Autodesk Fusion 360 part; units mm, degrees
note: some values were not read from the file. Set by a fixed rule: which sketch regions a step uses.
(part 46 of 59)
  spline S74 degree 5 poles (30.2174, 19.4214) (30.2148, 19.4218) (30.2094, 19.4225) (30.2014, 19.4236) (30.1907, 19.425) (30.1773, 19.4267) (30.164, 19.4284) (30.1507, 19.4301) (30.1375, 19.4317) (30.1242, 19.4334) (30.111, 19.435) (30.0979, 19.4366) (30.0847, 19.4382) (30.0716, 19.4398) (30.0585, 19.4413) (30.0455, 19.4428) (30.0324, 19.4443) (30.0194, 19.4458) (30.0065, 19.4473) (29.9935, 19.4487) (29.9806, 19.4501) (29.9678, 19.4516) (29.9549, 19.4529) (29.9421, 19.4543) (29.9293, 19.4556) (29.9166, 19.457) (29.9039, 19.4583) (29.8912, 19.4596) (29.8785, 19.4608) (29.8659, 19.4621) (29.8533, 19.4633) (29.8407, 19.4645) (29.8282, 19.4657) (29.8157, 19.4669) (29.8032, 19.468) (29.7908, 19.4691) (29.7784, 19.4702) (29.766, 19.4713) (29.7537, 19.4724) (29.7414, 19.4735) (29.7291, 19.4745) (29.7169, 19.4755) (29.7047, 19.4765) (29.6925, 19.4775) (29.6803, 19.4784) (29.6682, 19.4794) (29.6562, 19.4803) (29.6441, 19.4812) (29.6321, 19.4821) (29.6201, 19.483) (29.6082, 19.4838) (29.5963, 19.4846) (29.5844, 19.4855) (29.5726, 19.4863) (29.5608, 19.487) (29.549, 19.4878) (29.5373, 19.4885) (29.5256, 19.4892) (29.514, 19.49) (29.5023, 19.4906) (29.4907, 19.4913) (29.4792, 19.492) (29.4677, 19.4926) (29.4562, 19.4932) (29.4447, 19.4938) (29.4333, 19.4944) (29.422, 19.495) (29.4106, 19.4955) (29.3993, 19.496) (29.3881, 19.4965) (29.3768, 19.497) (29.3657, 19.4975) (29.3545, 19.498) (29.3434, 19.4984) (29.3323, 19.4989) (29.3213, 19.4993) (29.3103, 19.4997) (29.2993, 19.5001) (29.2884, 19.5004) (29.2775, 19.5008) (29.2667, 19.5011) (29.2559, 19.5014) (29.2451, 19.5017) (29.2344, 19.502) (29.2237, 19.5023) (29.213, 19.5025) (29.2024, 19.5028) (29.1919, 19.503) (29.1813, 19.5032) (29.1708, 19.5034) (29.1604, 19.5035) (29.15, 19.5037) (29.1396, 19.5038) (29.1293, 19.504) (29.119, 19.5041) (29.1088, 19.5042) (29.0986, 19.5043) (29.0884, 19.5043) (29.0783, 19.5044) (29.0682, 19.5044) (29.0582, 19.5045) (29.0482, 19.5045) (29.0383, 19.5045) (29.0284, 19.5045) (29.0185, 19.5044) (29.0087, 19.5044) (28.9989, 19.5043) (28.9892, 19.5043) (28.9795, 19.5042) (28.9698, 19.5041) (28.9602, 19.504) (28.9507, 19.5038) (28.9412, 19.5037) (28.9317, 19.5036) (28.9223, 19.5034) (28.9129, 19.5032) (28.9036, 19.503) (28.8943, 19.5028) (28.8851, 19.5026) (28.8759, 19.5024) (28.8668, 19.5021) (28.8577, 19.5019) (28.8486, 19.5016) (28.8396, 19.5014) (28.8307, 19.5011) (28.8218, 19.5008) (28.8129, 19.5005) (28.8041, 19.5001) (28.7953, 19.4998) (28.7866, 19.4995) (28.778, 19.4991) (28.7694, 19.4987) (28.7608, 19.4984) (28.7523, 19.498) (28.7438, 19.4976) (28.7354, 19.4972) (28.727, 19.4968) (28.7187, 19.4963) (28.7105, 19.4959) (28.7023, 19.4954) (28.6941, 19.495) (28.686, 19.4945) (28.678, 19.494) (28.67, 19.4936) (28.662, 19.4931) (28.6541, 19.4926) (28.6463, 19.4921) (28.6385, 19.4915) (28.6307, 19.491) (28.6231, 19.4905) (28.6154, 19.4899) (28.6079, 19.4894) (28.6004, 19.4888) (28.5929, 19.4882) (28.5855, 19.4877) (28.5781, 19.4871) (28.5709, 19.4865) (28.5636, 19.4859) (28.5564, 19.4853) (28.5493, 19.4847) (28.5423, 19.4841) (28.5353, 19.4835) (28.5283, 19.4828) (28.5214, 19.4822) (28.5146, 19.4816) (28.5078, 19.4809) (28.5011, 19.4803) (28.4945, 19.4796) (28.4879, 19.4789) (28.4814, 19.4783) (28.4749, 19.4776) (28.4685, 19.4769) (28.4622, 19.4763) (28.4559, 19.4756) (28.4497, 19.4749) (28.4435, 19.4742) (28.4374, 19.4735) (28.4314, 19.4728) (28.4255, 19.4721) (28.4196, 19.4714) (28.4137, 19.4707) (28.408, 19.47) (28.4023, 19.4693) (28.3966, 19.4686) (28.3911, 19.4679) (28.3856, 19.4672) (28.3802, 19.4665) (28.3748, 19.4658) (28.3695, 19.4651) (28.3643, 19.4644) (28.3592, 19.4637) (28.3541, 19.463) (28.3491, 19.4623) (28.3442, 19.4616) (28.3393, 19.4609) (28.3345, 19.4602) (28.3298, 19.4595) (28.3252, 19.4588) (28.3206, 19.4581) (28.3161, 19.4574) (28.3117, 19.4568) (28.3074, 19.4561) (28.3031, 19.4554) (28.2989, 19.4547) (28.2948, 19.4541) (28.2908, 19.4534) (28.2868, 19.4528) (28.283, 19.4521) (28.2792, 19.4515) (28.2755, 19.4508) (28.2719, 19.4502) (28.2683, 19.4496) (28.2649, 19.449) (28.2615, 19.4484) (28.2582, 19.4478) (28.255, 19.4472) (28.2519, 19.4466) (28.2489, 19.4461) (28.246, 19.4455) (28.2431, 19.445) (28.2404, 19.4445) (28.2377, 19.4439) (28.2351, 19.4434) (28.2327, 19.4429) (28.2303, 19.4425) (28.228, 19.442) (28.2258, 19.4416) (28.2237, 19.4411) (28.2217, 19.4407) (28.2198, 19.4403) (28.218, 19.4399) (28.2163, 19.4396) (28.2147, 19.4392) (28.2132, 19.4389) (28.2118, 19.4386) (28.2106, 19.4383) (28.2094, 19.4381) (28.2083, 19.4378) (28.2074, 19.4376) (28.2065, 19.4374) (28.2058, 19.4372) (28.2053, 19.4371) (28.205, 19.437) (28.2048, 19.437) (28.2047, 19.437) knots -1 -1 -1 -1 -1 -1 -0.99583333 -0.99166667 -0.9875 -0.98333333 -0.97916667 -0.975 -0.97083333 -0.96666667 -0.9625 -0.95833333 -0.95416667 -0.95 -0.94583333 -0.94166667 -0.9375 -0.93333333 -0.92916667 -0.925 -0.92083333 -0.91666667 -0.9125 -0.90833333 -0.90416667 -0.9 -0.89583333 -0.89166667 -0.8875 -0.88333333 -0.87916667 -0.875 -0.87083333 -0.86666667 -0.8625 -0.85833333 -0.85416667 -0.85 -0.84583333 -0.84166667 -0.8375 -0.83333333 -0.82916667 -0.825 -0.82083333 -0.81666667 -0.8125 -0.80833333 -0.80416667 -0.8 -0.79583333 -0.79166667 -0.7875 -0.78333333 -0.77916667 -0.775 -0.77083333 -0.76666667 -0.7625 -0.75833333 -0.75416667 -0.75 -0.74583333 -0.74166667 -0.7375 -0.73333333 -0.72916667 -0.725 -0.72083333 -0.71666667 -0.7125 -0.70833333 -0.70416667 -0.7 -0.69583333 -0.69166667 -0.6875 -0.68333333 -0.67916667 -0.675 -0.67083333 -0.66666667 -0.6625 -0.65833333 -0.65416667 -0.65 -0.64583333 -0.64166667 -0.6375 -0.63333333 -0.62916667 -0.625 -0.62083333 -0.61666667 -0.6125 -0.60833333 -0.60416667 -0.6 -0.59583333 -0.59166667 -0.5875 -0.58333333 -0.57916667 -0.575 -0.57083333 -0.56666667 -0.5625 -0.55833333 -0.55416667 -0.55 -0.54583333 -0.54166667 -0.5375 -0.53333333 -0.52916667 -0.525 -0.52083333 -0.51666667 -0.5125 -0.50833333 -0.50416667 -0.5 -0.49583333 -0.49166667 -0.4875 -0.48333333 -0.47916667 -0.475 -0.47083333 -0.46666667 -0.4625 -0.45833333 -0.45416667 -0.45 -0.44583333 -0.44166667 -0.4375 -0.43333333 -0.42916667 -0.425 -0.42083333 -0.41666667 -0.4125 -0.40833333 -0.40416667 -0.4 -0.39583333 -0.39166667 -0.3875 -0.38333333 -0.37916667 -0.375 -0.37083333 -0.36666667 -0.3625 -0.35833333 -0.35416667 -0.35 -0.34583333 -0.34166667 -0.3375 -0.33333333 -0.32916667 -0.325 -0.32083333 -0.31666667 -0.3125 -0.30833333 -0.30416667 -0.3 -0.29583333 -0.29166667 -0.2875 -0.28333333 -0.27916667 -0.275 -0.27083333 -0.26666667 -0.2625 -0.25833333 -0.25416667 -0.25 -0.24583333 -0.24166667 -0.2375 -0.23333333 -0.22916667 -0.225 -0.22083333 -0.21666667 -0.2125 -0.20833333 -0.20416667 -0.2 -0.19583333 -0.19166667 -0.1875 -0.18333333 -0.17916667 -0.175 -0.17083333 -0.16666667 -0.1625 -0.15833333 -0.15416667 -0.15 -0.14583333 -0.14166667 -0.1375 -0.13333333 -0.12916667 -0.125 -0.12083333 -0.11666667 -0.1125 -0.10833333 -0.10416667 -0.1 -0.09583333 -0.09166667 -0.0875 -0.08333333 -0.07916667 -0.075 -0.07083333 -0.06666667 -0.0625 -0.05833333 -0.05416667 -0.05 -0.04583333 -0.04166667 -0.0375 -0.03333333 -0.02916667 -0.025 -0.02083333 -0.01666667 -0.0125 -0.00833333 -0.00416667 0 0 0 0 0 0
  line L165 (28.2047, 19.437) -> (28.2039, 19.4368)
  line L166 (28.2039, 19.4368) -> (27.918, 19.3665)
  arc A75 (27.918, 19.3665) -> (27.6109, 20.5125) centre (0, 12.5) ccw
  line L167 (27.6109, 20.5125) -> (27.8937, 20.5945)
  line L168 (27.8937, 20.5945) -> (27.8945, 20.5948)
  spline S75 degree 5 poles (27.8945, 20.5948) (27.8946, 20.5948) (27.8948, 20.5948) (27.8951, 20.5949) (27.8956, 20.5951) (27.8963, 20.5953) (27.8971, 20.5956) (27.898, 20.5958) (27.8991, 20.5962) (27.9002, 20.5965) (27.9015, 20.5969) (27.9028, 20.5973) (27.9043, 20.5978) (27.9058, 20.5983) (27.9075, 20.5988) (27.9092, 20.5994) (27.9111, 20.6) (27.913, 20.6007) (27.915, 20.6013) (27.9172, 20.602) (27.9194, 20.6028) (27.9217, 20.6036) (27.9241, 20.6044) (27.9265, 20.6052) (27.9291, 20.6061) (27.9318, 20.607) (27.9345, 20.608) (27.9373, 20.609) (27.9402, 20.61) (27.9432, 20.6111) (27.9462, 20.6121) (27.9494, 20.6133) (27.9526, 20.6144) (27.9559, 20.6156) (27.9593, 20.6169) (27.9627, 20.6181) (27.9662, 20.6194) (27.9698, 20.6208) (27.9735, 20.6222) (27.9772, 20.6236) (27.9811, 20.625) (27.9849, 20.6265) (27.9889, 20.628) (27.9929, 20.6295) (27.997, 20.6311) (28.0012, 20.6327) (28.0054, 20.6344) (28.0097, 20.6361) (28.0141, 20.6378) (28.0185, 20.6395) (28.023, 20.6413) (28.0276, 20.6432) (28.0322, 20.645) (28.0369, 20.6469) (28.0416, 20.6488) (28.0464, 20.6508) (28.0513, 20.6528) (28.0562, 20.6548) (28.0612, 20.6569) (28.0663, 20.659) (28.0714, 20.6611) (28.0765, 20.6633) (28.0818, 20.6655) (28.087, 20.6677) (28.0924, 20.67) (28.0978, 20.6723) (28.1032, 20.6747) (28.1087, 20.677) (28.1143, 20.6795) (28.1199, 20.6819) (28.1256, 20.6844) (28.1313, 20.6869) (28.1371, 20.6895) (28.1429, 20.692) (28.1488, 20.6947) (28.1547, 20.6973) (28.1607, 20.7) (28.1667, 20.7027) (28.1728, 20.7055) (28.179, 20.7083) (28.1851, 20.7111) (28.1914, 20.714) (28.1977, 20.7169) (28.204, 20.7198) (28.2104, 20.7227) (28.2168, 20.7257) (28.2233, 20.7288) (28.2298, 20.7318) (28.2363, 20.7349) (28.2429, 20.7381) (28.2496, 20.7412) (28.2563, 20.7445) (28.263, 20.7477) (28.2698, 20.751) (28.2767, 20.7543) (28.2835, 20.7576) (28.2905, 20.761) (28.2974, 20.7644) (28.3044, 20.7678) (28.3115, 20.7713) (28.3186, 20.7748) (28.3257, 20.7784) (28.3329, 20.782) (28.3401, 20.7856) (28.3473, 20.7892) (28.3546, 20.7929) (28.3619, 20.7966) (28.3693, 20.8004) (28.3767, 20.8042) (28.3842, 20.808) (28.3917, 20.8118) (28.3992, 20.8157) (28.4068, 20.8196) (28.4144, 20.8236) (28.422, 20.8276) (28.4297, 20.8316) (28.4374, 20.8357) (28.4452, 20.8398) (28.4529, 20.8439) (28.4608, 20.848) (28.4686, 20.8522) (28.4765, 20.8565) (28.4845, 20.8607) (28.4924, 20.865) (28.5004, 20.8693) (28.5085, 20.8737) (28.5165, 20.8781) (28.5246, 20.8825) (28.5328, 20.887) (28.5409, 20.8915) (28.5491, 20.896) (28.5574, 20.9006) (28.5657, 20.9052) (28.574, 20.9098) (28.5823, 20.9145) (28.5907, 20.9192) (28.5991, 20.9239) (28.6075, 20.9287) (28.616, 20.9335) (28.6244, 20.9384) (28.633, 20.9432) (28.6415, 20.9481) (28.6501, 20.9531) (28.6587, 20.958) (28.6674, 20.963) (28.676, 20.9681) (28.6847, 20.9732) (28.6935, 20.9783) (28.7022, 20.9834) (28.711, 20.9886) (28.7199, 20.9938) (28.7287, 20.999) (28.7376, 21.0043) (28.7465, 21.0096) (28.7554, 21.015) (28.7644, 21.0203) (28.7734, 21.0257) (28.7824, 21.0312) (28.7914, 21.0367) (28.8005, 21.0422) (28.8096, 21.0477) (28.8187, 21.0533) (28.8279, 21.0589) (28.837, 21.0645) (28.8462, 21.0702) (28.8555, 21.0759) (28.8647, 21.0817) (28.874, 21.0874) (28.8833, 21.0932) (28.8926, 21.0991) (28.902, 21.105) (28.9113, 21.1109) (28.9207, 21.1168) (28.9302, 21.1228) (28.9396, 21.1288) (28.9491, 21.1348) (28.9586, 21.1409) (28.9681, 21.147) (28.9776, 21.1532) (28.9872, 21.1593) (28.9968, 21.1656) (29.0064, 21.1718) (29.016, 21.1781) (29.0257, 21.1844) (29.0354, 21.1907) (29.0451, 21.1971) (29.0548, 21.2035) (29.0646, 21.2099) (29.0743, 21.2164) (29.0841, 21.2229) (29.0939, 21.2295) (29.1037, 21.236) (29.1136, 21.2426) (29.1235, 21.2493) (29.1334, 21.2559) (29.1433, 21.2626) (29.1532, 21.2694) (29.1632, 21.2762) (29.1731, 21.283) (29.1831, 21.2898) (29.1932, 21.2967) (29.2032, 21.3036) (29.2132, 21.3105) (29.2233, 21.3175) (29.2334, 21.3245) (29.2435, 21.3315) (29.2537, 21.3386) (29.2638, 21.3457) (29.274, 21.3528) (29.2842, 21.36) (29.2944, 21.3671) (29.3046, 21.3744) (29.3148, 21.3816) (29.3251, 21.3889) (29.3354, 21.3963) (29.3457, 21.4036) (29.356, 21.411) (29.3663, 21.4184) (29.3766, 21.4259) (29.387, 21.4334) (29.3974, 21.4409) (29.4078, 21.4485) (29.4182, 21.456) (29.4286, 21.4637) (29.4391, 21.4713) (29.4495, 21.479) (29.46, 21.4867) (29.4705, 21.4945) (29.481, 21.5022) (29.4915, 21.5101) (29.5021, 21.5179) (29.5127, 21.5258) (29.5232, 21.5337) (29.5338, 21.5416) (29.5444, 21.5496) (29.555, 21.5576) (29.5657, 21.5657) (29.5763, 21.5737) (29.587, 21.5818) (29.5977, 21.59) (29.6084, 21.5981) (29.6169, 21.6047) (29.6234, 21.6096) (29.6276, 21.6129) (29.6298, 21.6146) knots 0 0 0 0 0 0 0.00416667 0.00833333 0.0125 0.01666667 0.02083333 0.025 0.02916667 0.03333333 0.0375 0.04166667 0.04583333 0.05 0.05416667 0.05833333 0.0625 0.06666667 0.07083333 0.075 0.07916667 0.08333333 0.0875 0.09166667 0.09583333 0.1 0.10416667 0.10833333 0.1125 0.11666667 0.12083333 0.125 0.12916667 0.13333333 0.1375 0.14166667 0.14583333 0.15 0.15416667 0.15833333 0.1625 0.16666667 0.17083333 0.175 0.17916667 0.18333333 0.1875 0.19166667 0.19583333 0.2 0.20416667 0.20833333 0.2125 0.21666667 0.22083333 0.225 0.22916667 0.23333333 0.2375 0.24166667 0.24583333 0.25 0.25416667 0.25833333 0.2625 0.26666667 0.27083333 0.275 0.27916667 0.28333333 0.2875 0.29166667 0.29583333 0.3 0.30416667 0.30833333 0.3125 0.31666667 0.32083333 0.325 0.32916667 0.33333333 0.3375 0.34166667 0.34583333 0.35 0.35416667 0.35833333 0.3625 0.36666667 0.37083333 0.375 0.37916667 0.38333333 0.3875 0.39166667 0.39583333 0.4 0.40416667 0.40833333 0.4125 0.41666667 0.42083333 0.425 0.42916667 0.43333333 0.4375 0.44166667 0.44583333 0.45 0.45416667 0.45833333 0.4625 0.46666667 0.47083333 0.475 0.47916667 0.48333333 0.4875 0.49166667 0.49583333 0.5 0.50416667 0.50833333 0.5125 0.51666667 0.52083333 0.525 0.52916667 0.53333333 0.5375 0.54166667 0.54583333 0.55 0.55416667 0.55833333 0.5625 0.56666667 0.57083333 0.575 0.57916667 0.58333333 0.5875 0.59166667 0.59583333 0.6 0.60416667 0.60833333 0.6125 0.61666667 0.62083333 0.625 0.62916667 0.63333333 0.6375 0.64166667 0.64583333 0.65 0.65416667 0.65833333 0.6625 0.66666667 0.67083333 0.675 0.67916667 0.68333333 0.6875 0.69166667 0.69583333 0.7 0.70416667 0.70833333 0.7125 0.71666667 0.72083333 0.725 0.72916667 0.73333333 0.7375 0.74166667 0.74583333 0.75 0.75416667 0.75833333 0.7625 0.76666667 0.77083333 0.775 0.77916667 0.78333333 0.7875 0.79166667 0.79583333 0.8 0.80416667 0.80833333 0.8125 0.81666667 0.82083333 0.825 0.82916667 0.83333333 0.8375 0.84166667 0.84583333 0.85 0.85416667 0.85833333 0.8625 0.86666667 0.87083333 0.875 0.87916667 0.88333333 0.8875 0.89166667 0.89583333 0.9 0.90416667 0.90833333 0.9125 0.91666667 0.92083333 0.925 0.92916667 0.93333333 0.9375 0.94166667 0.94583333 0.95 0.95416667 0.95833333 0.9625 0.96666667 0.97083333 0.975 0.97916667 0.98333333 0.9875 0.99166667 0.99583333 1 1 1 1 1 1
  arc A76 (29.6298, 21.6146) -> (29.3284, 22.5421) centre (0, 12.5) ccw
  line L169 (26.6221, 23.3547) -> (26.8948, 23.4659)
  line L170 (26.8948, 23.4659) -> (26.8955, 23.4662)
  spline S76 degree 5 poles (26.8955, 23.4662) (26.8956, 23.4662) (26.8958, 23.4663) (26.8961, 23.4664) (26.8966, 23.4666) (26.8973, 23.4669) (26.8981, 23.4672) (26.899, 23.4676) (26.9, 23.4681) (26.9011, 23.4685) (26.9023, 23.4691) (26.9036, 23.4696) (26.905, 23.4702) (26.9065, 23.4709) (26.908, 23.4716) (26.9097, 23.4724) (26.9115, 23.4731) (26.9134, 23.474) (26.9153, 23.4749) (26.9173, 23.4758) (26.9195, 23.4768) (26.9217, 23.4778) (26.924, 23.4788) (26.9263, 23.4799) (26.9288, 23.4811) (26.9313, 23.4823) (26.9339, 23.4835) (26.9366, 23.4848) (26.9394, 23.4861) (26.9423, 23.4875) (26.9452, 23.4889) (26.9482, 23.4903) (26.9513, 23.4918) (26.9544, 23.4934) (26.9577, 23.4949) (26.961, 23.4966) (26.9643, 23.4982) (26.9678, 23.4999) (26.9713, 23.5017) (26.9748, 23.5035) (26.9785, 23.5053) (26.9822, 23.5072) (26.986, 23.5091) (26.9898, 23.5111) (26.9937, 23.5131) (26.9977, 23.5151) (27.0017, 23.5172) (27.0058, 23.5193) (27.01, 23.5215) (27.0142, 23.5237) (27.0185, 23.5259) (27.0228, 23.5282) (27.0272, 23.5306) (27.0317, 23.5329) (27.0362, 23.5353) (27.0408, 23.5378) (27.0454, 23.5403) (27.0501, 23.5428) (27.0549, 23.5454) (27.0597, 23.548) (27.0645, 23.5507) (27.0694, 23.5534) (27.0744, 23.5561) (27.0794, 23.5589) (27.0845, 23.5617) (27.0896, 23.5646) (27.0948, 23.5675) (27.1, 23.5704) (27.1053, 23.5734) (27.1106, 23.5764) (27.116, 23.5795) (27.1214, 23.5826) (27.1269, 23.5857) (27.1324, 23.5889) (27.138, 23.5921) (27.1436, 23.5954) (27.1493, 23.5987) (27.155, 23.602) (27.1608, 23.6054) (27.1666, 23.6088) (27.1725, 23.6123) (27.1784, 23.6158) (27.1843, 23.6193) (27.1903, 23.6229) (27.1963, 23.6265) (27.2024, 23.6301) (27.2085, 23.6338) (27.2147, 23.6376) (27.2209, 23.6413) (27.2271, 23.6451) (27.2334, 23.649) (27.2397, 23.6529) (27.2461, 23.6568) (27.2525, 23.6608) (27.259, 23.6648) (27.2654, 23.6688) (27.272, 23.6729) (27.2785, 23.677) (27.2851, 23.6812) (27.2918, 23.6854) (27.2985, 23.6896) (27.3052, 23.6939) (27.3119, 23.6982) (27.3187, 23.7025) (27.3256, 23.7069) (27.3324, 23.7113) (27.3393, 23.7158) (27.3463, 23.7203) (27.3533, 23.7248) (27.3603, 23.7294) (27.3673, 23.734) (27.3744, 23.7387) (27.3815, 23.7434) (27.3887, 23.7481) (27.3958, 23.7529) (27.4031, 23.7577) (27.4103, 23.7625) (27.4176, 23.7674) (27.4249, 23.7723) (27.4323, 23.7773) (27.4396, 23.7823) (27.447, 23.7873) (27.4545, 23.7924) (27.462, 23.7975) (27.4695, 23.8026) (27.477, 23.8078) (27.4846, 23.813) (27.4922, 23.8183) (27.4998, 23.8235) (27.5074, 23.8289) (27.5151, 23.8342) (27.5228, 23.8396) (27.5306, 23.8451) (27.5384, 23.8506) (27.5462, 23.8561) (27.554, 23.8616) (27.5618, 23.8672) (27.5697, 23.8728) (27.5776, 23.8785) (27.5856, 23.8842) (27.5936, 23.8899) (27.6015, 23.8957) (27.6096, 23.9015) (27.6176, 23.9074) (27.6257, 23.9132) (27.6338, 23.9192) (27.6419, 23.9251) (27.6501, 23.9311) (27.6582, 23.9371) (27.6665, 23.9432) (27.6747, 23.9493) (27.6829, 23.9554) (27.6912, 23.9616) (27.6995, 23.9678) (27.7078, 23.9741) (27.7162, 23.9803) (27.7246, 23.9867) (27.733, 23.993) (27.7414, 23.9994) (27.7498, 24.0058) (27.7583, 24.0123) (27.7668, 24.0188) (27.7753, 24.0253) (27.7838, 24.0319) (27.7924, 24.0385) (27.801, 24.0452) (27.8096, 24.0518) (27.8182, 24.0585) (27.8268, 24.0653) (27.8355, 24.0721) (27.8442, 24.0789) (27.8529, 24.0858) (27.8616, 24.0927) (27.8704, 24.0996) (27.8791, 24.1065) (27.8879, 24.1135) (27.8967, 24.1206) (27.9055, 24.1276) (27.9144, 24.1348) (27.9233, 24.1419) (27.9322, 24.1491) (27.9411, 24.1563) (27.95, 24.1635) (27.9589, 24.1708) (27.9679, 24.1781) (27.9769, 24.1855) (27.9859, 24.1929) (27.9949, 24.2003) (28.0039, 24.2078) (28.013, 24.2153) (28.0221, 24.2228) (28.0312, 24.2303) (28.0403, 24.2379) (28.0494, 24.2456) (28.0585, 24.2532) (28.0677, 24.2609) (28.0769, 24.2687) (28.0861, 24.2765) (28.0953, 24.2843) (28.1045, 24.2921) (28.1137, 24.3) (28.123, 24.3079) (28.1323, 24.3158) (28.1416, 24.3238) (28.1509, 24.3318) (28.1602, 24.3399) (28.1695, 24.348) (28.1789, 24.3561) (28.1882, 24.3643) (28.1976, 24.3724) (28.207, 24.3807) (28.2164, 24.3889) (28.2259, 24.3972) (28.2353, 24.4055) (28.2447, 24.4139) (28.2542, 24.4223) (28.2637, 24.4307) (28.2732, 24.4392) (28.2827, 24.4477) (28.2922, 24.4562) (28.3018, 24.4648) (28.3113, 24.4734) (28.3209, 24.482) (28.3305, 24.4907) (28.34, 24.4994) (28.3496, 24.5081) (28.3593, 24.5169) (28.3689, 24.5257) (28.3785, 24.5345) (28.3882, 24.5434) (28.3978, 24.5523) (28.4075, 24.5613) (28.4172, 24.5702) (28.4269, 24.5792) (28.4366, 24.5883) (28.4464, 24.5973) (28.4561, 24.6065) (28.4658, 24.6156) (28.4756, 24.6248) (28.4854, 24.634) (28.4951, 24.6432) (28.503, 24.6506) (28.5089, 24.6562) (28.5128, 24.66) (28.5147, 24.6618) knots 0 0 0 0 0 0 0.00416667 0.00833333 0.0125 0.01666667 0.02083333 0.025 0.02916667 0.03333333 0.0375 0.04166667 0.04583333 0.05 0.05416667 0.05833333 0.0625 0.06666667 0.07083333 0.075 0.07916667 0.08333333 0.0875 0.09166667 0.09583333 0.1 0.10416667 0.10833333 0.1125 0.11666667 0.12083333 0.125 0.12916667 0.13333333 0.1375 0.14166667 0.14583333 0.15 0.15416667 0.15833333 0.1625 0.16666667 0.17083333 0.175 0.17916667 0.18333333 0.1875 0.19166667 0.19583333 0.2 0.20416667 0.20833333 0.2125 0.21666667 0.22083333 0.225 0.22916667 0.23333333 0.2375 0.24166667 0.24583333 0.25 0.25416667 0.25833333 0.2625 0.26666667 0.27083333 0.275 0.27916667 0.28333333 0.2875 0.29166667 0.29583333 0.3 0.30416667 0.30833333 0.3125 0.31666667 0.32083333 0.325 0.32916667 0.33333333 0.3375 0.34166667 0.34583333 0.35 0.35416667 0.35833333 0.3625 0.36666667 0.37083333 0.375 0.37916667 0.38333333 0.3875 0.39166667 0.39583333 0.4 0.40416667 0.40833333 0.4125 0.41666667 0.42083333 0.425 0.42916667 0.43333333 0.4375 0.44166667 0.44583333 0.45 0.45416667 0.45833333 0.4625 0.46666667 0.47083333 0.475 0.47916667 0.48333333 0.4875 0.49166667 0.49583333 0.5 0.50416667 0.50833333 0.5125 0.51666667 0.52083333 0.525 0.52916667 0.53333333 0.5375 0.54166667 0.54583333 0.55 0.55416667 0.55833333 0.5625 0.56666667 0.57083333 0.575 0.57916667 0.58333333 0.5875 0.59166667 0.59583333 0.6 0.60416667 0.60833333 0.6125 0.61666667 0.62083333 0.625 0.62916667 0.63333333 0.6375 0.64166667 0.64583333 0.65 0.65416667 0.65833333 0.6625 0.66666667 0.67083333 0.675 0.67916667 0.68333333 0.6875 0.69166667 0.69583333 0.7 0.70416667 0.70833333 0.7125 0.71666667 0.72083333 0.725 0.72916667 0.73333333 0.7375 0.74166667 0.74583333 0.75 0.75416667 0.75833333 0.7625 0.76666667 0.77083333 0.775 0.77916667 0.78333333 0.7875 0.79166667 0.79583333 0.8 0.80416667 0.80833333 0.8125 0.81666667 0.82083333 0.825 0.82916667 0.83333333 0.8375 0.84166667 0.84583333 0.85 0.85416667 0.85833333 0.8625 0.86666667 0.87083333 0.875 0.87916667 0.88333333 0.8875 0.89166667 0.89583333 0.9 0.90416667 0.90833333 0.9125 0.91666667 0.92083333 0.925 0.92916667 0.93333333 0.9375 0.94166667 0.94583333 0.95 0.95416667 0.95833333 0.9625 0.96666667 0.97083333 0.975 0.97916667 0.98333333 0.9875 0.99166667 0.99583333 1 1 1 1 1 1
  arc A77 (28.5147, 24.6618) -> (28.1181, 25.5527) centre (0, 12.5) ccw
  spline S77 degree 5 poles (28.1181, 25.5527) (28.1154, 25.5525) (28.11, 25.5521) (28.1019, 25.5515) (28.0911, 25.5506) (28.0777, 25.5495) (28.0644, 25.5484) (28.051, 25.5473) (28.0377, 25.5462) (28.0244, 25.5451) (28.0112, 25.5439) (27.9979, 25.5427) (27.9848, 25.5415) (27.9716, 25.5404) (27.9585, 25.5391) (27.9454, 25.5379) (27.9323, 25.5367) (27.9193, 25.5354) (27.9063, 25.5342) (27.8934, 25.5329) (27.8805, 25.5316) (27.8676, 25.5303) (27.8547, 25.529) (27.8419, 25.5276) (27.8291, 25.5263) (27.8164, 25.5249) (27.8037, 25.5236) (27.791, 25.5222) (27.7784, 25.5208) (27.7658, 25.5194) (27.7532, 25.518) (27.7406, 25.5165) (27.7281, 25.5151) (27.7157, 25.5136) (27.7032, 25.5122) (27.6908, 25.5107) (27.6785, 25.5092) (27.6661, 25.5077) (27.6539, 25.5062) (27.6416, 25.5047) (27.6294, 25.5031) (27.6172, 25.5016) (27.605, 25.5) (27.5929, 25.4984) (27.5809, 25.4968) (27.5688, 25.4952) (27.5568, 25.4936) (27.5449, 25.492) (27.5329, 25.4904) (27.521, 25.4887) (27.5092, 25.4871) (27.4974, 25.4854) (27.4856, 25.4838) (27.4738, 25.4821) (27.4621, 25.4804) (27.4505, 25.4787) (27.4388, 25.477) (27.4273, 25.4752) (27.4157, 25.4735) (27.4042, 25.4718) (27.3927, 25.47) (27.3813, 25.4682) (27.3699, 25.4665) (27.3585, 25.4647) (27.3472, 25.4629) (27.3359, 25.4611) (27.3247, 25.4593) (27.3135, 25.4574) (27.3023, 25.4556) (27.2912, 25.4538) (27.2801, 25.4519) (27.2691, 25.4501) (27.2581, 25.4482) (27.2471, 25.4463) (27.2362, 25.4445) (27.2253, 25.4426) (27.2145, 25.4407) (27.2037, 25.4388) (27.1929, 25.4368) (27.1822, 25.4349) (27.1715, 25.433) (27.1609, 25.4311) (27.1503, 25.4291) (27.1397, 25.4272) (27.1292, 25.4252) (27.1188, 25.4232) (27.1083, 25.4213) (27.0979, 25.4193) (27.0876, 25.4173) (27.0773, 25.4153) (27.0671, 25.4133) (27.0568, 25.4113) (27.0467, 25.4093) (27.0365, 25.4072) (27.0265, 25.4052) (27.0164, 25.4032) (27.0064, 25.4011) (26.9965, 25.3991) (26.9866, 25.3971) (26.9767, 25.395) (26.9669, 25.3929) (26.9571, 25.3909) (26.9474, 25.3888) (26.9377, 25.3867) (26.9281, 25.3847) (26.9185, 25.3826) (26.9089, 25.3805) (26.8994, 25.3784) (26.89, 25.3763) (26.8806, 25.3742) (26.8712, 25.3721) (26.8619, 25.37) (26.8526, 25.3679) (26.8434, 25.3658) (26.8342, 25.3636) (26.8251, 25.3615) (26.816, 25.3594) (26.8069, 25.3573) (26.798, 25.3551) (26.789, 25.353) (26.7801, 25.3509) (26.7713, 25.3487) (26.7625, 25.3466) (26.7537, 25.3445) (26.7451, 25.3423) (26.7364, 25.3402) (26.7278, 25.338) (26.7193, 25.3359) (26.7108, 25.3337) (26.7023, 25.3316) (26.6939, 25.3294) (26.6856, 25.3273) (26.6773, 25.3251) (26.669, 25.323) (26.6608, 25.3208) (26.6527, 25.3187) (26.6446, 25.3166) (26.6365, 25.3144) (26.6286, 25.3123) (26.6206, 25.3101) (26.6127, 25.308) (26.6049, 25.3058) (26.5971, 25.3037) (26.5894, 25.3016) (26.5817, 25.2994) (26.5741, 25.2973) (26.5665, 25.2952) (26.559, 25.293) (26.5516, 25.2909) (26.5442, 25.2888) (26.5368, 25.2867) (26.5296, 25.2845) (26.5223, 25.2824) (26.5151, 25.2803) (26.508, 25.2782) (26.5009, 25.2761) (26.4939, 25.274) (26.487, 25.272) (26.4801, 25.2699) (26.4733, 25.2678) (26.4665, 25.2657) (26.4598, 25.2637) (26.4531, 25.2616) (26.4465, 25.2596) (26.4399, 25.2575) (26.4335, 25.2555) (26.427, 25.2534) (26.4207, 25.2514) (26.4144, 25.2494) (26.4081, 25.2474) (26.4019, 25.2454) (26.3958, 25.2434) (26.3897, 25.2414) (26.3837, 25.2395) (26.3778, 25.2375) (26.3719, 25.2356) (26.3661, 25.2336) (26.3604, 25.2317) (26.3547, 25.2298) (26.3491, 25.2279) (26.3435, 25.226) (26.338, 25.2241) (26.3326, 25.2222) (26.3273, 25.2204) (26.322, 25.2185) (26.3167, 25.2167) (26.3116, 25.2149) (26.3065, 25.2131) (26.3015, 25.2113) (26.2965, 25.2095) (26.2916, 25.2077) (26.2868, 25.206) (26.282, 25.2043) (26.2774, 25.2026) (26.2728, 25.2009) (26.2682, 25.1992) (26.2638, 25.1975) (26.2594, 25.1959) (26.255, 25.1943) (26.2508, 25.1927) (26.2466, 25.1911) (26.2425, 25.1895) (26.2385, 25.188) (26.2345, 25.1864) (26.2307, 25.1849) (26.2269, 25.1834) (26.2231, 25.182) (26.2195, 25.1806) (26.2159, 25.1791) (26.2124, 25.1778) (26.209, 25.1764) (26.2057, 25.175) (26.2024, 25.1737) (26.1993, 25.1724) (26.1962, 25.1712) (26.1932, 25.1699) (26.1903, 25.1687) (26.1874, 25.1676) (26.1847, 25.1664) (26.182, 25.1653) (26.1794, 25.1642) (26.1769, 25.1631) (26.1745, 25.1621) (26.1722, 25.1611) (26.17, 25.1602) (26.1678, 25.1592) (26.1658, 25.1583) (26.1638, 25.1575) (26.1619, 25.1567) (26.1602, 25.1559) (26.1585, 25.1551) (26.1569, 25.1544) (26.1554, 25.1538) (26.154, 25.1531) (26.1527, 25.1526) (26.1515, 25.152) (26.1504, 25.1515) (26.1495, 25.151) (26.1486, 25.1506) (26.1478, 25.1503) (26.1471, 25.15) (26.1467, 25.1497) (26.1464, 25.1496) (26.1462, 25.1495) (26.1461, 25.1495) knots -1 -1 -1 -1 -1 -1 -0.99583333 -0.99166667 -0.9875 -0.98333333 -0.97916667 -0.975 -0.97083333 -0.96666667 -0.9625 -0.95833333 -0.95416667 -0.95 -0.94583333 -0.94166667 -0.9375 -0.93333333 -0.92916667 -0.925 -0.92083333 -0.91666667 -0.9125 -0.90833333 -0.90416667 -0.9 -0.89583333 -0.89166667 -0.8875 -0.88333333 -0.87916667 -0.875 -0.87083333 -0.86666667 -0.8625 -0.85833333 -0.85416667 -0.85 -0.84583333 -0.84166667 -0.8375 -0.83333333 -0.82916667 -0.825 -0.82083333 -0.81666667 -0.8125 -0.80833333 -0.80416667 -0.8 -0.79583333 -0.79166667 -0.7875 -0.78333333 -0.77916667 -0.775 -0.77083333 -0.76666667 -0.7625 -0.75833333 -0.75416667 -0.75 -0.74583333 -0.74166667 -0.7375 -0.73333333 -0.72916667 -0.725 -0.72083333 -0.71666667 -0.7125 -0.70833333 -0.70416667 -0.7 -0.69583333 -0.69166667 -0.6875 -0.68333333 -0.67916667 -0.675 -0.67083333 -0.66666667 -0.6625 -0.65833333 -0.65416667 -0.65 -0.64583333 -0.64166667 -0.6375 -0.63333333 -0.62916667 -0.625 -0.62083333 -0.61666667 -0.6125 -0.60833333 -0.60416667 -0.6 -0.59583333 -0.59166667 -0.5875 -0.58333333 -0.57916667 -0.575 -0.57083333 -0.56666667 -0.5625 -0.55833333 -0.55416667 -0.55 -0.54583333 -0.54166667 -0.5375 -0.53333333 -0.52916667 -0.525 -0.52083333 -0.51666667 -0.5125 -0.50833333 -0.50416667 -0.5 -0.49583333 -0.49166667 -0.4875 -0.48333333 -0.47916667 -0.475 -0.47083333 -0.46666667 -0.4625 -0.45833333 -0.45416667 -0.45 -0.44583333 -0.44166667 -0.4375 -0.43333333 -0.42916667 -0.425 -0.42083333 -0.41666667 -0.4125 -0.40833333 -0.40416667 -0.4 -0.39583333 -0.39166667 -0.3875 -0.38333333 -0.37916667 -0.375 -0.37083333 -0.36666667 -0.3625 -0.35833333 -0.35416667 -0.35 -0.34583333 -0.34166667 -0.3375 -0.33333333 -0.32916667 -0.325 -0.32083333 -0.31666667 -0.3125 -0.30833333 -0.30416667 -0.3 -0.29583333 -0.29166667 -0.2875 -0.28333333 -0.27916667 -0.275 -0.27083333 -0.26666667 -0.2625 -0.25833333 -0.25416667 -0.25 -0.24583333 -0.24166667 -0.2375 -0.23333333 -0.22916667 -0.225 -0.22083333 -0.21666667 -0.2125 -0.20833333 -0.20416667 -0.2 -0.19583333 -0.19166667 -0.1875 -0.18333333 -0.17916667 -0.175 -0.17083333 -0.16666667 -0.1625 -0.15833333 -0.15416667 -0.15 -0.14583333 -0.14166667 -0.1375 -0.13333333 -0.12916667 -0.125 -0.12083333 -0.11666667 -0.1125 -0.10833333 -0.10416667 -0.1 -0.09583333 -0.09166667 -0.0875 -0.08333333 -0.07916667 -0.075 -0.07083333 -0.06666667 -0.0625 -0.05833333 -0.05416667 -0.05 -0.04583333 -0.04166667 -0.0375 -0.03333333 -0.02916667 -0.025 -0.02083333 -0.01666667 -0.0125 -0.00833333 -0.00416667 0 0 0 0 0 0
  line L171 (26.1461, 25.1495) -> (26.1453, 25.1491)
  line L172 (26.1453, 25.1491) -> (25.8803, 25.0209)
  dimension "d110" = 10
  dimension "d111" = 10
  constraint horizontal L149
  constraint vertical L150
  constraint horizontal L151
  constraint vertical L152
  constraint coincident L6.end L7.start
  constraint horizontal L153
  constraint vertical L154
  constraint horizontal L155
  constraint vertical L156
  constraint coincident L2.end L3.start
  measures "d110" distance of L6.end L151.end
  measures "d111" distance of L2.end L155.end
extrude "押し出し16" add sketch "スケッチ22" against normal blind 8 contours L2 L153 L154 L155 L156 | L6 L149 L150 L151 L152
sketch "スケッチ23" plane through (0, -19, 0) normal (0, -1, 0) x (1, 0, 0)
  circle A0 centre (0, 30) radius 1.7
  line L0 (-4, 25) -> (4, 25)
  line L1 (4, 25) -> (4, 45)
  line L2 (4, 45) -> (-4, 45)
  line L3 (-4, 45) -> (-4, 25)
  line L4 (0, 45) -> (0, 40)
  circle A1 centre (0, 40) radius 1.6
  circle A2 centre (0, 30) radius 1.6
  dimension "d114" = 5
  dimension "d115" = 3.2
  dimension "d116" = 3.2
  constraint midpoint L2 L4.start
  constraint perpendicular L2 L4
  constraint coincident L4.end A1.centre
  constraint concentric A0 A2
  measures "d114" distance of L4.start L4.end
  measures "d115" diameter of A1
  measures "d116" diameter of A2
extrude "押し出し17" cut sketch "スケッチ23" against normal blind 38 contours A1
extrude "押し出し18" add sketch "スケッチ23" against normal blind 8 contours A0
sketch "スケッチ24" plane through (0, 19, 0) normal (0, 1, 0) x (-1, 0, 0)
  circle A0 centre (0, 40) radius 1.6
  circle A1 centre (0, 30) radius 1.7
  line L0 (-4, 25) -> (4, 25)
  line L1 (4, 25) -> (4, 45)
  line L2 (4, 45) -> (-4, 45)
  line L3 (-4, 45) -> (-4, 25)
  circle A2 centre (0, 30) radius 1.6
  dimension "d121" = 3.2
  constraint concentric A1 A2
  measures "d121" diameter of A2
extrude "押し出し19" add sketch "スケッチ24" against normal blind 8 contours A1
sketch "スケッチ25" plane through (4, 0, 0) normal (1, 0, 0) x (0, 1, 0)
  circle A0 centre (0, 12.5) radius 4
  line L0 (-19, 25) -> (-25.8803, 25.0209)
  line L1 (-25.8803, 25.0209) -> (-26.1453, 25.1491)
  line L2 (-26.1453, 25.1491) -> (-26.1461, 25.1495)
  spline S0 degree 5 poles (-26.1461, 25.1495) (-26.1462, 25.1495) (-26.1464, 25.1496) (-26.1467, 25.1497) (-26.1471, 25.15) (-26.1478, 25.1503) (-26.1486, 25.1506) (-26.1495, 25.151) (-26.1504, 25.1515) (-26.1515, 25.152) (-26.1527, 25.1526) (-26.154, 25.1531) (-26.1554, 25.1538) (-26.1569, 25.1544) (-26.1585, 25.1551) (-26.1602, 25.1559) (-26.1619, 25.1567) (-26.1638, 25.1575) (-26.1658, 25.1583) (-26.1678, 25.1592) (-26.17, 25.1602) (-26.1722, 25.1611) (-26.1745, 25.1621) (-26.1769, 25.1631) (-26.1794, 25.1642) (-26.182, 25.1653) (-26.1847, 25.1664) (-26.1874, 25.1676) (-26.1903, 25.1687) (-26.1932, 25.1699) (-26.1962, 25.1712) (-26.1993, 25.1724) (-26.2024, 25.1737) (-26.2057, 25.175) (-26.209, 25.1764) (-26.2124, 25.1778) (-26.2159, 25.1791) (-26.2195, 25.1806) (-26.2231, 25.182) (-26.2269, 25.1834) (-26.2307, 25.1849) (-26.2345, 25.1864) (-26.2385, 25.188) (-26.2425, 25.1895) (-26.2466, 25.1911) (-26.2508, 25.1927) (-26.255, 25.1943) (-26.2594, 25.1959) (-26.2638, 25.1975) (-26.2682, 25.1992) (-26.2728, 25.2009) (-26.2774, 25.2026) (-26.282, 25.2043) (-26.2868, 25.206) (-26.2916, 25.2077) (-26.2965, 25.2095) (-26.3015, 25.2113) (-26.3065, 25.2131) (-26.3116, 25.2149) (-26.3167, 25.2167) (-26.322, 25.2185) (-26.3273, 25.2204) (-26.3326, 25.2222) (-26.338, 25.2241) (-26.3435, 25.226) (-26.3491, 25.2279) (-26.3547, 25.2298) (-26.3604, 25.2317) (-26.3661, 25.2336) (-26.3719, 25.2356) (-26.3778, 25.2375) (-26.3837, 25.2395) (-26.3897, 25.2414) (-26.3958, 25.2434) (-26.4019, 25.2454) (-26.4081, 25.2474) (-26.4144, 25.2494) (-26.4207, 25.2514) (-26.427, 25.2534) (-26.4335, 25.2555) (-26.4399, 25.2575) (-26.4465, 25.2596) (-26.4531, 25.2616) (-26.4598, 25.2637) (-26.4665, 25.2657) (-26.4733, 25.2678) (-26.4801, 25.2699) (-26.487, 25.272) (-26.4939, 25.274) (-26.5009, 25.2761) (-26.508, 25.2782) (-26.5151, 25.2803) (-26.5223, 25.2824) (-26.5296, 25.2845) (-26.5368, 25.2867) (-26.5442, 25.2888) (-26.5516, 25.2909) (-26.559, 25.293) (-26.5665, 25.2952) (-26.5741, 25.2973) (-26.5817, 25.2994) (-26.5894, 25.3016) (-26.5971, 25.3037) (-26.6049, 25.3058) (-26.6127, 25.308) (-26.6206, 25.3101) (-26.6286, 25.3123) (-26.6365, 25.3144) (-26.6446, 25.3166) (-26.6527, 25.3187) (-26.6608, 25.3208) (-26.669, 25.323) (-26.6773, 25.3251) (-26.6856, 25.3273) (-26.6939, 25.3294) (-26.7023, 25.3316) (-26.7108, 25.3337) (-26.7193, 25.3359) (-26.7278, 25.338) (-26.7364, 25.3402) (-26.7451, 25.3423) (-26.7537, 25.3445) (-26.7625, 25.3466) (-26.7713, 25.3487) (-26.7801, 25.3509) (-26.789, 25.353) (-26.798, 25.3551) (-26.8069, 25.3573) (-26.816, 25.3594) (-26.8251, 25.3615) (-26.8342, 25.3636) (-26.8434, 25.3658) (-26.8526, 25.3679) (-26.8619, 25.37) (-26.8712, 25.3721) (-26.8806, 25.3742) (-26.89, 25.3763) (-26.8994, 25.3784) (-26.9089, 25.3805) (-26.9185, 25.3826) (-26.9281, 25.3847) (-26.9377, 25.3867) (-26.9474, 25.3888) (-26.9571, 25.3909) (-26.9669, 25.3929) (-26.9767, 25.395) (-26.9866, 25.3971) (-26.9965, 25.3991) (-27.0064, 25.4011) (-27.0164, 25.4032) (-27.0265, 25.4052) (-27.0365, 25.4072) (-27.0467, 25.4093) (-27.0568, 25.4113) (-27.0671, 25.4133) (-27.0773, 25.4153) (-27.0876, 25.4173) (-27.0979, 25.4193) (-27.1083, 25.4213) (-27.1188, 25.4232) (-27.1292, 25.4252) (-27.1397, 25.4272) (-27.1503, 25.4291) (-27.1609, 25.4311) (-27.1715, 25.433) (-27.1822, 25.4349) (-27.1929, 25.4368) (-27.2037, 25.4388) (-27.2145, 25.4407) (-27.2253, 25.4426) (-27.2362, 25.4445) (-27.2471, 25.4463) (-27.2581, 25.4482) (-27.2691, 25.4501) (-27.2801, 25.4519) (-27.2912, 25.4538) (-27.3023, 25.4556) (-27.3135, 25.4574) (-27.3247, 25.4593) (-27.3359, 25.4611) (-27.3472, 25.4629) (-27.3585, 25.4647) (-27.3699, 25.4665) (-27.3813, 25.4682) (-27.3927, 25.47) (-27.4042, 25.4718) (-27.4157, 25.4735) (-27.4273, 25.4752) (-27.4388, 25.477) (-27.4505, 25.4787) (-27.4621, 25.4804) (-27.4738, 25.4821) (-27.4856, 25.4838) (-27.4974, 25.4854) (-27.5092, 25.4871) (-27.521, 25.4887) (-27.5329, 25.4904) (-27.5449, 25.492) (-27.5568, 25.4936) (-27.5688, 25.4952) (-27.5809, 25.4968) (-27.5929, 25.4984) (-27.605, 25.5) (-27.6172, 25.5016) (-27.6294, 25.5031) (-27.6416, 25.5047) (-27.6539, 25.5062) (-27.6661, 25.5077) (-27.6785, 25.5092) (-27.6908, 25.5107) (-27.7032, 25.5122) (-27.7157, 25.5136) (-27.7281, 25.5151) (-27.7406, 25.5165) (-27.7532, 25.518) (-27.7658, 25.5194) (-27.7784, 25.5208) (-27.791, 25.5222) (-27.8037, 25.5236) (-27.8164, 25.5249) (-27.8291, 25.5263) (-27.8419, 25.5276) (-27.8547, 25.529) (-27.8676, 25.5303) (-27.8805, 25.5316) (-27.8934, 25.5329) (-27.9063, 25.5342) (-27.9193, 25.5354) (-27.9323, 25.5367) (-27.9454, 25.5379) (-27.9585, 25.5391) (-27.9716, 25.5404) (-27.9848, 25.5415) (-27.9979, 25.5427) (-28.0112, 25.5439) (-28.0244, 25.5451) (-28.0377, 25.5462) (-28.051, 25.5473) (-28.0644, 25.5484) (-28.0777, 25.5495) (-28.0911, 25.5506) (-28.1019, 25.5515) (-28.11, 25.5521) (-28.1154, 25.5525) (-28.1181, 25.5527) knots 0 0 0 0 0 0 0.00416667 0.00833333 0.0125 0.01666667 0.02083333 0.025 0.02916667 0.03333333 0.0375 0.04166667 0.04583333 0.05 0.05416667 0.05833333 0.0625 0.06666667 0.07083333 0.075 0.07916667 0.08333333 0.0875 0.09166667 0.09583333 0.1 0.10416667 0.10833333 0.1125 0.11666667 0.12083333 0.125 0.12916667 0.13333333 0.1375 0.14166667 0.14583333 0.15 0.15416667 0.15833333 0.1625 0.16666667 0.17083333 0.175 0.17916667 0.18333333 0.1875 0.19166667 0.19583333 0.2 0.20416667 0.20833333 0.2125 0.21666667 0.22083333 0.225 0.22916667 0.23333333 0.2375 0.24166667 0.24583333 0.25 0.25416667 0.25833333 0.2625 0.26666667 0.27083333 0.275 0.27916667 0.28333333 0.2875 0.29166667 0.29583333 0.3 0.30416667 0.30833333 0.3125 0.31666667 0.32083333 0.325 0.32916667 0.33333333 0.3375 0.34166667 0.34583333 0.35 0.35416667 0.35833333 0.3625 0.36666667 0.37083333 0.375 0.37916667 0.38333333 0.3875 0.39166667 0.39583333 0.4 0.40416667 0.40833333 0.4125 0.41666667 0.42083333 0.425 0.42916667 0.43333333 0.4375 0.44166667 0.44583333 0.45 0.45416667 0.45833333 0.4625 0.46666667 0.47083333 0.475 0.47916667 0.48333333 0.4875 0.49166667 0.49583333 0.5 0.50416667 0.50833333 0.5125 0.51666667 0.52083333 0.525 0.52916667 0.53333333 0.5375 0.54166667 0.54583333 0.55 0.55416667 0.55833333 0.5625 0.56666667 0.57083333 0.575 0.57916667 0.58333333 0.5875 0.59166667 0.59583333 0.6 0.60416667 0.60833333 0.6125 0.61666667 0.62083333 0.625 0.62916667 0.63333333 0.6375 0.64166667 0.64583333 0.65 0.65416667 0.65833333 0.6625 0.66666667 0.67083333 0.675 0.67916667 0.68333333 0.6875 0.69166667 0.69583333 0.7 0.70416667 0.70833333 0.7125 0.71666667 0.72083333 0.725 0.72916667 0.73333333 0.7375 0.74166667 0.74583333 0.75 0.75416667 0.75833333 0.7625 0.76666667 0.77083333 0.775 0.77916667 0.78333333 0.7875 0.79166667 0.79583333 0.8 0.80416667 0.80833333 0.8125 0.81666667 0.82083333 0.825 0.82916667 0.83333333 0.8375 0.84166667 0.84583333 0.85 0.85416667 0.85833333 0.8625 0.86666667 0.87083333 0.875 0.87916667 0.88333333 0.8875 0.89166667 0.89583333 0.9 0.90416667 0.90833333 0.9125 0.91666667 0.92083333 0.925 0.92916667 0.93333333 0.9375 0.94166667 0.94583333 0.95 0.95416667 0.95833333 0.9625 0.96666667 0.97083333 0.975 0.97916667 0.98333333 0.9875 0.99166667 0.99583333 1 1 1 1 1 1
  arc A1 (-28.1181, 25.5527) -> (-28.5147, 24.6618) centre (0, 12.5) ccw
  spline S1 degree 5 poles (-28.5147, 24.6618) (-28.5128, 24.66) (-28.5089, 24.6562) (-28.503, 24.6506) (-28.4951, 24.6432) (-28.4854, 24.634) (-28.4756, 24.6248) (-28.4658, 24.6156) (-28.4561, 24.6065) (-28.4464, 24.5973) (-28.4366, 24.5883) (-28.4269, 24.5792) (-28.4172, 24.5702) (-28.4075, 24.5613) (-28.3978, 24.5523) (-28.3882, 24.5434) (-28.3785, 24.5345) (-28.3689, 24.5257) (-28.3593, 24.5169) (-28.3496, 24.5081) (-28.34, 24.4994) (-28.3305, 24.4907) (-28.3209, 24.482) (-28.3113, 24.4734) (-28.3018, 24.4648) (-28.2922, 24.4562) (-28.2827, 24.4477) (-28.2732, 24.4392) (-28.2637, 24.4307) (-28.2542, 24.4223) (-28.2447, 24.4139) (-28.2353, 24.4055) (-28.2259, 24.3972) (-28.2164, 24.3889) (-28.207, 24.3807) (-28.1976, 24.3724) (-28.1882, 24.3643) (-28.1789, 24.3561) (-28.1695, 24.348) (-28.1602, 24.3399) (-28.1509, 24.3318) (-28.1416, 24.3238) (-28.1323, 24.3158) (-28.123, 24.3079) (-28.1137, 24.3) (-28.1045, 24.2921) (-28.0953, 24.2843) (-28.0861, 24.2765) (-28.0769, 24.2687) (-28.0677, 24.2609) (-28.0585, 24.2532) (-28.0494, 24.2456) (-28.0403, 24.2379) (-28.0312, 24.2303) (-28.0221, 24.2228) (-28.013, 24.2153) (-28.0039, 24.2078) (-27.9949, 24.2003) (-27.9859, 24.1929) (-27.9769, 24.1855) (-27.9679, 24.1781) (-27.9589, 24.1708) (-27.95, 24.1635) (-27.9411, 24.1563) (-27.9322, 24.1491) (-27.9233, 24.1419) (-27.9144, 24.1348) (-27.9055, 24.1276) (-27.8967, 24.1206) (-27.8879, 24.1135) (-27.8791, 24.1065) (-27.8704, 24.0996) (-27.8616, 24.0927) (-27.8529, 24.0858) (-27.8442, 24.0789) (-27.8355, 24.0721) (-27.8268, 24.0653) (-27.8182, 24.0585) (-27.8096, 24.0518) (-27.801, 24.0452) (-27.7924, 24.0385) (-27.7838, 24.0319) (-27.7753, 24.0253) (-27.7668, 24.0188) (-27.7583, 24.0123) (-27.7498, 24.0058) (-27.7414, 23.9994) (-27.733, 23.993) (-27.7246, 23.9867) (-27.7162, 23.9803) (-27.7078, 23.9741) (-27.6995, 23.9678) (-27.6912, 23.9616) (-27.6829, 23.9554) (-27.6747, 23.9493) (-27.6665, 23.9432) (-27.6582, 23.9371) (-27.6501, 23.9311) (-27.6419, 23.9251) (-27.6338, 23.9192) (-27.6257, 23.9132) (-27.6176, 23.9074) (-27.6096, 23.9015) (-27.6015, 23.8957) (-27.5936, 23.8899) (-27.5856, 23.8842) (-27.5776, 23.8785) (-27.5697, 23.8728) (-27.5618, 23.8672) (-27.554, 23.8616) (-27.5462, 23.8561) (-27.5384, 23.8506) (-27.5306, 23.8451) (-27.5228, 23.8396) (-27.5151, 23.8342) (-27.5074, 23.8289) (-27.4998, 23.8235) (-27.4922, 23.8183) (-27.4846, 23.813) (-27.477, 23.8078) (-27.4695, 23.8026) (-27.462, 23.7975) (-27.4545, 23.7924) (-27.447, 23.7873) (-27.4396, 23.7823) (-27.4323, 23.7773) (-27.4249, 23.7723) (-27.4176, 23.7674) (-27.4103, 23.7625) (-27.4031, 23.7577) (-27.3958, 23.7529) (-27.3887, 23.7481) (-27.3815, 23.7434) (-27.3744, 23.7387) (-27.3673, 23.734) (-27.3603, 23.7294) (-27.3533, 23.7248) (-27.3463, 23.7203) (-27.3393, 23.7158) (-27.3324, 23.7113) (-27.3256, 23.7069) (-27.3187, 23.7025) (-27.3119, 23.6982) (-27.3052, 23.6939) (-27.2985, 23.6896) (-27.2918, 23.6854) (-27.2851, 23.6812) (-27.2785, 23.677) (-27.272, 23.6729) (-27.2654, 23.6688) (-27.259, 23.6648) (-27.2525, 23.6608) (-27.2461, 23.6568) (-27.2397, 23.6529) (-27.2334, 23.649) (-27.2271, 23.6451) (-27.2209, 23.6413) (-27.2147, 23.6376) (-27.2085, 23.6338) (-27.2024, 23.6301) (-27.1963, 23.6265) (-27.1903, 23.6229) (-27.1843, 23.6193) (-27.1784, 23.6158) (-27.1725, 23.6123) (-27.1666, 23.6088) (-27.1608, 23.6054) (-27.155, 23.602) (-27.1493, 23.5987) (-27.1436, 23.5954) (-27.138, 23.5921) (-27.1324, 23.5889) (-27.1269, 23.5857) (-27.1214, 23.5826) (-27.116, 23.5795) (-27.1106, 23.5764) (-27.1053, 23.5734) (-27.1, 23.5704) (-27.0948, 23.5675) (-27.0896, 23.5646) (-27.0845, 23.5617) (-27.0794, 23.5589) (-27.0744, 23.5561) (-27.0694, 23.5534) (-27.0645, 23.5507) (-27.0597, 23.548) (-27.0549, 23.5454) (-27.0501, 23.5428) (-27.0454, 23.5403) (-27.0408, 23.5378) (-27.0362, 23.5353) (-27.0317, 23.5329) (-27.0272, 23.5306) (-27.0228, 23.5282) (-27.0185, 23.5259) (-27.0142, 23.5237) (-27.01, 23.5215) (-27.0058, 23.5193) (-27.0017, 23.5172) (-26.9977, 23.5151) (-26.9937, 23.5131) (-26.9898, 23.5111) (-26.986, 23.5091) (-26.9822, 23.5072) (-26.9785, 23.5053) (-26.9748, 23.5035) (-26.9713, 23.5017) (-26.9678, 23.4999) (-26.9643, 23.4982) (-26.961, 23.4966) (-26.9577, 23.4949) (-26.9544, 23.4934) (-26.9513, 23.4918) (-26.9482, 23.4903) (-26.9452, 23.4889) (-26.9423, 23.4875) (-26.9394, 23.4861) (-26.9366, 23.4848) (-26.9339, 23.4835) (-26.9313, 23.4823) (-26.9288, 23.4811) (-26.9263, 23.4799) (-26.924, 23.4788) (-26.9217, 23.4778) (-26.9195, 23.4768) (-26.9173, 23.4758) (-26.9153, 23.4749) (-26.9134, 23.474) (-26.9115, 23.4731) (-26.9097, 23.4724) (-26.908, 23.4716) (-26.9065, 23.4709) (-26.905, 23.4702) (-26.9036, 23.4696) (-26.9023, 23.4691) (-26.9011, 23.4685) (-26.9, 23.4681) (-26.899, 23.4676) (-26.8981, 23.4672) (-26.8973, 23.4669) (-26.8966, 23.4666) (-26.8961, 23.4664) (-26.8958, 23.4663) (-26.8956, 23.4662) (-26.8955, 23.4662) knots -1 -1 -1 -1 -1 -1 -0.99583333 -0.99166667 -0.9875 -0.98333333 -0.97916667 -0.975 -0.97083333 -0.96666667 -0.9625 -0.95833333 -0.95416667 -0.95 -0.94583333 -0.94166667 -0.9375 -0.93333333 -0.92916667 -0.925 -0.92083333 -0.91666667 -0.9125 -0.90833333 -0.90416667 -0.9 -0.89583333 -0.89166667 -0.8875 -0.88333333 -0.87916667 -0.875 -0.87083333 -0.86666667 -0.8625 -0.85833333 -0.85416667 -0.85 -0.84583333 -0.84166667 -0.8375 -0.83333333 -0.82916667 -0.825 -0.82083333 -0.81666667 -0.8125 -0.80833333 -0.80416667 -0.8 -0.79583333 -0.79166667 -0.7875 -0.78333333 -0.77916667 -0.775 -0.77083333 -0.76666667 -0.7625 -0.75833333 -0.75416667 -0.75 -0.74583333 -0.74166667 -0.7375 -0.73333333 -0.72916667 -0.725 -0.72083333 -0.71666667 -0.7125 -0.70833333 -0.70416667 -0.7 -0.69583333 -0.69166667 -0.6875 -0.68333333 -0.67916667 -0.675 -0.67083333 -0.66666667 -0.6625 -0.65833333 -0.65416667 -0.65 -0.64583333 -0.64166667 -0.6375 -0.63333333 -0.62916667 -0.625 -0.62083333 -0.61666667 -0.6125 -0.60833333 -0.60416667 -0.6 -0.59583333 -0.59166667 -0.5875 -0.58333333 -0.57916667 -0.575 -0.57083333 -0.56666667 -0.5625 -0.55833333 -0.55416667 -0.55 -0.54583333 -0.54166667 -0.5375 -0.53333333 -0.52916667 -0.525 -0.52083333 -0.51666667 -0.5125 -0.50833333 -0.50416667 -0.5 -0.49583333 -0.49166667 -0.4875 -0.48333333 -0.47916667 -0.475 -0.47083333 -0.46666667 -0.4625 -0.45833333 -0.45416667 -0.45 -0.44583333 -0.44166667 -0.4375 -0.43333333 -0.42916667 -0.425 -0.42083333 -0.41666667 -0.4125 -0.40833333 -0.40416667 -0.4 -0.39583333 -0.39166667 -0.3875 -0.38333333 -0.37916667 -0.375 -0.37083333 -0.36666667 -0.3625 -0.35833333 -0.35416667 -0.35 -0.34583333 -0.34166667 -0.3375 -0.33333333 -0.32916667 -0.325 -0.32083333 -0.31666667 -0.3125 -0.30833333 -0.30416667 -0.3 -0.29583333 -0.29166667 -0.2875 -0.28333333 -0.27916667 -0.275 -0.27083333 -0.26666667 -0.2625 -0.25833333 -0.25416667 -0.25 -0.24583333 -0.24166667 -0.2375 -0.23333333 -0.22916667 -0.225 -0.22083333 -0.21666667 -0.2125 -0.20833333 -0.20416667 -0.2 -0.19583333 -0.19166667 -0.1875 -0.18333333 -0.17916667 -0.175 -0.17083333 -0.16666667 -0.1625 -0.15833333 -0.15416667 -0.15 -0.14583333 -0.14166667 -0.1375 -0.13333333 -0.12916667 -0.125 -0.12083333 -0.11666667 -0.1125 -0.10833333 -0.10416667 -0.1 -0.09583333 -0.09166667 -0.0875 -0.08333333 -0.07916667 -0.075 -0.07083333 -0.06666667 -0.0625 -0.05833333 -0.05416667 -0.05 -0.04583333 -0.04166667 -0.0375 -0.03333333 -0.02916667 -0.025 -0.02083333 -0.01666667 -0.0125 -0.00833333 -0.00416667 0 0 0 0 0 0
  line L3 (-26.8955, 23.4662) -> (-26.8948, 23.4659)
  line L4 (-26.8948, 23.4659) -> (-26.6221, 23.3547)
  arc A2 (-26.6221, 23.3547) -> (-27.0473, 22.2471) centre (0, 12.5) ccw
  line L5 (-27.0473, 22.2471) -> (-27.3243, 22.3469)
  line L6 (-27.3243, 22.3469) -> (-27.3251, 22.3472)